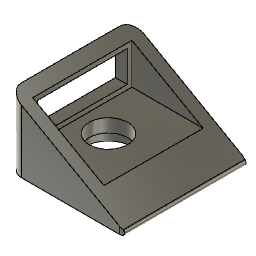
WaterLevel_Top v7 (Autodesk Fusion 360 design; units mm, degrees)
Autodesk Fusion 360 part; units mm, degrees
sketch "Sketch1" plane through (0, 0, 0) normal (0, 0, 1) x (1, 0, 0)
  line L0 (0, 0) -> (130, 0)
  line L1 (130, 0) -> (130, 130)
  line L2 (130, 130) -> (0, 130)
  line L3 (0, 130) -> (0, 0)
  dimension "d1" = 130
  dimension "d2" = 130
  constraint horizontal L0
  constraint vertical L1
  constraint horizontal L2
  constraint vertical L3
  constraint coincident L0.start L3.end
  measures "d1" distance of L1.end L2.end
  measures "d2" distance of L0.start L2.end
extrude "Extrude1" add sketch "Sketch1" along normal blind 74
sketch "Sketch2" plane through (0, 0, 74) normal (0, 0, 1) x (-1, 0, 0)
  line L0 (0, -130) -> (0, 0)
  line L1 (0, 0) -> (-130, 0)
  line L2 (-130, 0) -> (-130, -130)
  line L3 (-130, -130) -> (0, -130)
  line L4 (-12.5, -117.5) -> (-117.5, -117.5)
  line L5 (-117.5, -117.5) -> (-117.5, -12.5)
  line L6 (-117.5, -12.5) -> (-12.5, -12.5)
  line L7 (-12.5, -12.5) -> (-12.5, -117.5)
  line L8 (-75, -130) -> (-75, -117.5) construction
  line L9 (-75, 0) -> (-75, -12.5) construction
  line L10 (0, -65) -> (-12.5, -65) construction
  line L11 (-117.5, -65) -> (-130, -65) construction
  dimension "d5" = 12.5
  constraint horizontal L4
  constraint vertical L5
  constraint horizontal L6
  constraint vertical L7
  constraint coincident L3 L8.start
  constraint coincident L4 L8.end
  constraint vertical L8
  constraint coincident L1 L9.start
  constraint coincident L6 L9.end
  constraint perpendicular L6 L9
  constraint coincident L0 L10.start
  constraint midpoint L7 L10.end
  constraint perpendicular L7 L10
  constraint coincident L5 L11.start
  constraint coincident L2 L11.end
  constraint perpendicular L2 L11
  constraint collinear L10 L11
  constraint collinear L8 L9
  constraint equal L9 L11
  constraint equal L10 L11
  constraint equal L8 L10
  measures "d5" distance of L8.start L8.end
extrude "Extrude2" cut sketch "Sketch2" against normal blind 50 contours L4 L5 L6 L7
sketch "Sketch3" plane through (0, 0, 24) normal (0, 0, 1) x (-1, 0, 0)
  line L0 (-12.5, -12.5) -> (-117.5, -12.5)
  line L1 (-117.5, -12.5) -> (-117.5, -117.5)
  line L2 (-117.5, -117.5) -> (-12.5, -117.5)
  line L3 (-12.5, -117.5) -> (-12.5, -12.5)
  line L4 (-12.5, -62.5893) -> (-42.5, -62.5893) construction
  line L5 (-42.5, -62.5893) -> (-42.5, -117.5) construction
  line L6 (-42.5, -62.5893) -> (-117.5, -62.5893) construction
  line L7 (-42.5, -62.5893) -> (-65, -12.5) construction
  circle A0 centre (-42.5, -62.5893) radius 20.447
  dimension "d8" = 40.894
  dimension "d25" = 30
  constraint coincident L3 L4.start
  constraint perpendicular L3 L4
  constraint coincident L2 L5.end
  constraint perpendicular L2 L5
  constraint coincident L1 L6.end
  constraint perpendicular L1 L6
  constraint midpoint L0 L7.end
  constraint equal L5 L7
  constraint coincident L4.end L5.start
  measures "d8" diameter of A0
  measures "d25" distance of L4.start L4.end
extrude "Extrude3" cut sketch "Sketch3" against normal through all contours A0
sketch "Sketch4" plane through (0, 0, 0) normal (0, 0, -1) x (1, 0, 0)
  circle A0 centre (42.5, -62.5893) radius 20.447
  line L0 (0, 0) -> (0, -130)
  line L1 (0, -130) -> (130, -130)
  line L2 (130, -130) -> (130, 0)
  line L3 (130, 0) -> (0, 0)
  circle A1 centre (42.5, -62.5893) radius 24.257
  dimension "d10" = 48.514
  constraint concentric A0 A1
  measures "d10" diameter of A1
extrude "Extrude4" cut sketch "Sketch4" against normal blind 10 contours A1
sketch "Sketch5" plane through (0, 0, 0) normal (0, -1, 0) x (1, 0, 0)
  line L0 (0, 0) -> (130, 0)
  line L1 (130, 0) -> (130, 74)
  line L2 (130, 74) -> (0, 74)
  line L3 (0, 74) -> (0, 0)
  line L4 (0, 74) -> (130, 0)
  line L5 (130, 74) -> (0, 74)
  line L6 (130, 74) -> (130, 0)
  constraint coincident L2.end L3.start
  constraint coincident L0.end L1.start
  constraint coincident L1.end L2.start
fillet "Fillet2" radius 13 4 edges at (130, 130, 37) (0, 130, 37) (130, 0, 37) (0, 0, 37)
extrude "Extrude5" cut sketch "Sketch5" against normal through all contours L1 L2 L4 L5 L6
sketch "Sketch6" plane through (12.5, 0, 0) normal (1, 0, 0) x (0, 1, 0)
  line L0 (117.5, 66.8846) -> (12.5, 66.8846)
  line L1 (12.5, 66.8846) -> (12.5, 24)
  line L2 (12.5, 24) -> (117.5, 24)
  line L3 (117.5, 24) -> (117.5, 66.8846)
  line L4 (17.5, 61.8846) -> (112.5, 61.8846)
  line L5 (112.5, 61.8846) -> (112.5, 29)
  line L6 (112.5, 29) -> (17.5, 29)
  line L7 (17.5, 29) -> (17.5, 61.8846)
  line L8 (108.6296, 61.8846) -> (108.6296, 66.8846) construction
  line L9 (112.5, 45.4423) -> (117.5, 45.4423) construction
  line L10 (108.6296, 29) -> (108.6296, 24) construction
  line L11 (12.5, 45.4423) -> (17.5, 45.4423) construction
  dimension "d18" = 5
  dimension "d19" = 5
  constraint horizontal L4
  constraint vertical L5
  constraint horizontal L6
  constraint vertical L7
  constraint coincident L4 L8.start
  constraint coincident L0 L8.end
  constraint perpendicular L0 L8
  constraint midpoint L5 L9.start
  constraint midpoint L3 L9.end
  constraint coincident L6 L10.start
  constraint coincident L2 L10.end
  constraint perpendicular L2 L10
  constraint collinear L8 L10
  constraint coincident L1 L11.start
  constraint coincident L7 L11.end
  constraint perpendicular L7 L11
  constraint collinear L9 L11
  constraint equal L9 L11
  measures "d18" distance of L8.start L8.end
  measures "d19" distance of L11.start L11.end
extrude "Extrude6" cut sketch "Sketch6" against normal through all contours L4 L5 L6 L7
fillet "Fillet3" radius 3 1 edges at (130, 65, 0)
